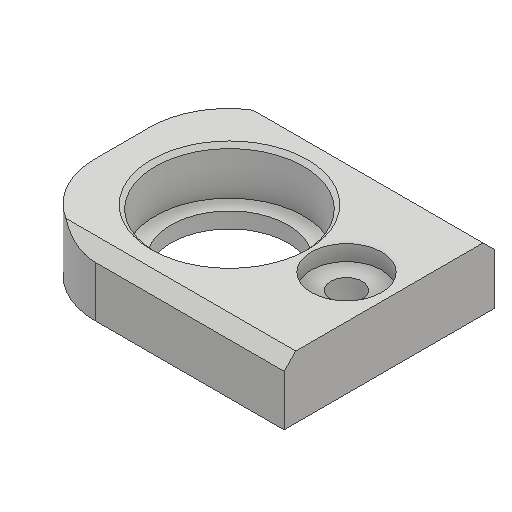
# Autodesk Inventor part: 3DP_ABS_Y_Axis_Pulley_Rod_Side_Bearing_Block
Saved by Autodesk Inventor 2026.1 (Build 301233000, 233)
## iProperties
Created: 2016-06-18
Part Number: 3DP_ABS_Y_Axis_Pulley_Rod_Side_Bearing_Block
Material: Ogólny
Document SubType Name: Modeling
Designer: Andrzej
Density: 1 g/cm^3
Appearance: Domyślna
Mass: 6.24318 g
Surface Area: 35.0559 cm^2
Volume: 6.24318 cm^3
Author: Andrzej
Autodesk Inventor part; units mm, degrees
ref_plane "YZ Plane" through (0, 0, 0) normal (1, 0, 0) x (0, 1, 0)
ref_plane "XZ Plane" through (0, 0, 0) normal (0, 1, 0) x (-1, 0, 0)
ref_plane "XY Plane" through (0, 0, 0) normal (0, 0, 1) x (1, 0, 0)
sketch "Szkic1" plane through (0, 0, 0) normal (0, 0, 1) x (1, 0, 0)
  line L0 (0.8088, 2.7684) -> (35.0088, 2.7684)
  line L1 (35.0088, 2.7684) -> (35.0088, -24.2316)
  line L2 (35.0088, -24.2316) -> (0.8088, -24.2316)
  line L3 (0.8088, -24.2316) -> (0.8088, 2.7684)
  circle A0 centre (14.5088, -10.7316) radius 9.5
  circle A1 centre (29.5088, -10.7316) radius 2
  circle A2 centre (14.5088, -10.7316) radius 7.5
  point P0 (0, 0)
  dimension "d0" = 34.2
  dimension "d1" = 27
  dimension "d2" = 13.5
  dimension "d3" = 20.5
  dimension "d4" = 19
  dimension "d5" = 13.5
  dimension "d7" = 4
  dimension "d11" = 5.5
  dimension "d14" = 13.5
  dimension "d15" = 2
  constraints: 8 end point, 3 centre point, 2 coincident, 2 parallel, 1 horizontal, 1 perpendicular
  measures "d0" distance of L1.end L2.end
  measures "d1" distance of L0.end L1.end
  measures "d2" distance from line of L0 point (14.509, -10.732)
  measures "d3" distance from line of L1 point (14.509, -10.732)
  measures "d4" diameter of A0
  measures "d5" distance from line of L0 A0.centre
  measures "d7" diameter of A1
  measures "d11" distance from line of L1 point (29.509, -10.732)
  measures "d14" distance from line of L0 point (29.509, -10.732)
  measures "d15" radial gap between concentric circles of A0 A2
extrude "Wyciągnięcie proste1" add sketch "Szkic1" along normal blind 8 contours L0 L1 L2 L3
extrude "Wyciągnięcie proste2" add sketch "Szkic1" along normal blind 2 contours A0
chamfer "Faza1" distance 0.5 angle 45 1 edges at (5.0088, -10.7316, 8)
chamfer "Faza2" distance 1.5 angle 45 2 edges at (17.9088, 2.7684, 8) (17.9088, -24.2316, 8)
sketch "Szkic2" plane through (0, 0, 8) normal (0, 0, 1) x (1, 0, 0)
  circle A0 centre (29.5088, -10.7316) radius 2 projected
  circle A1 centre (29.5088, -10.7316) radius 4.5
  point P0 (0, 0)
  dimension "d30" = 9
  constraints: 1 centre point, 1 coincident
  measures "d30" diameter of A1
extrude "Wyciągnięcie proste5" cut sketch "Szkic2" against normal blind 2
fillet "Zaokrąglenie1" radius 10 2 edges at (0.8088, -24.2316, 3.25) (0.8088, 2.7684, 3.25)
